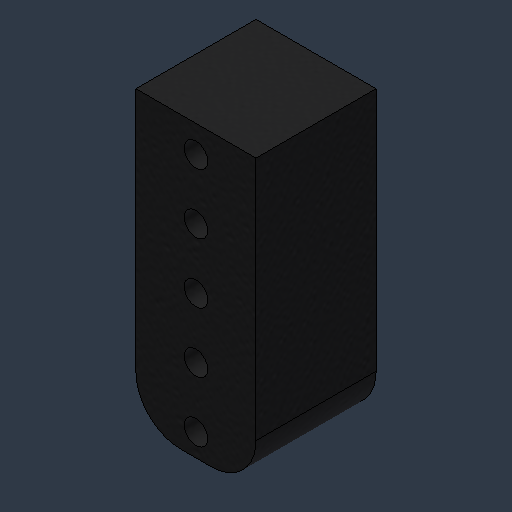
# Autodesk Inventor part: SDS LOWERING SPACER
Saved by Autodesk Inventor 2024.3 (Build 283343000, 343)
## iProperties
ILogicPurgeVersion: 0.0.0.0
OnSaveVersion: 3.5.0.0
OnSaveAssembly: COREAutomationManager
Category: _
Manager: _
Created: 2025-03-17
Part Number: SDS LOWERING SPACER
Checked By: 00
Engr Approved By: _
User Status: Work In Process
Material: Nylon 6/6
Description: STANDARD (mm)
Document SubType Name: Modeling
Mfg Approved By: John.Thibert
Designer: John.Thibert
Manufacturer: Standard
Standards Organization: Custom
Mass: 40.762 g
Surface Area: 90.2219 cm^2
Volume: 36.0726 cm^3
Density: 1.13 g/cm^3
Appearance: Black
CN_MASS: 0.04
CN_SERVICEABLE: _
FIRST_DESCRIPTION: _
SECOND_DESCRIPTION: _
THIRD_DESCRIPTION: _
ModelCat: Uncategorized
MaterialName: Nylon 6/6
Subject: _
Author: John.Thibert
Keywords: -
Revision Number: A
Autodesk Inventor part; units mm, degrees
ref_plane "YZ Plane" through (0, 0, 0) normal (1, 0, 0) x (0, 1, 0)
ref_plane "XZ Plane" through (0, 0, 0) normal (0, 1, 0) x (-1, 0, 0)
ref_plane "XY Plane" through (0, 0, 0) normal (0, 0, 1) x (1, 0, 0)
sketch "Sketch2" plane through (0, 0, 0) normal (0, 0, 1) x (1, 0, 0)
  line L0 (-12.7, -30.6388) -> (12.7, -30.6388)
  line L1 (12.7, -30.6388) -> (12.7, 30.6388)
  line L2 (12.7, 30.6388) -> (-12.7, 30.6388)
  line L3 (-12.7, 30.6388) -> (-12.7, -30.6388)
  line L4 (-12.7, -30.6388) -> (12.7, 30.6388) construction
  line L5 (12.7, -30.6388) -> (-12.7, 30.6388) construction
  line L6 (0, 30.6388) -> (0, -30.6388) construction
  point P0 (0, 0)
  dimension "d0" = 25.4
  dimension "d1" = 61.2775
  constraints: 14 end point, 4 midpoint, 2 parallel, 1 horizontal, 1 perpendicular
  measures "d0" distance of L2.end L1.end
  measures "d1" distance of L1.end L0.end
extrude "Extrusion1" add sketch "Sketch2" along normal blind 25.4
sketch "Sketch3" plane through (0, 0, 25.4) normal (0, 0, 1) x (1, 0, 0)
  line L0 (-12.7, -30.6388) -> (12.7, -30.6388) construction
  point P0 (0, 0)
  point P1 (0, -25.8762)
  dimension "d5" = 4.7625
  constraints: 1 vertical alignment
  measures "d5" distance from line of L0 point (0, -25.876)
hole "Hole1" at (0, -25.8762, 25.4) direction (0, 0, -1) diameter 4.9784 end through all start extended yes clearance for "Flat Head Machine Screw (82)" size "#10" standard "Ansi Unified Screw Threads"
fillet "Fillet1" radius 9.525 2 edges at (-12.7, -30.6388, 12.7) (12.7, -30.6388, 12.7)
pattern_linear "Rectangular Pattern1" count 5 spacing 12.7 along (0, 1, 0) of "Hole1"
body "Solid1"
